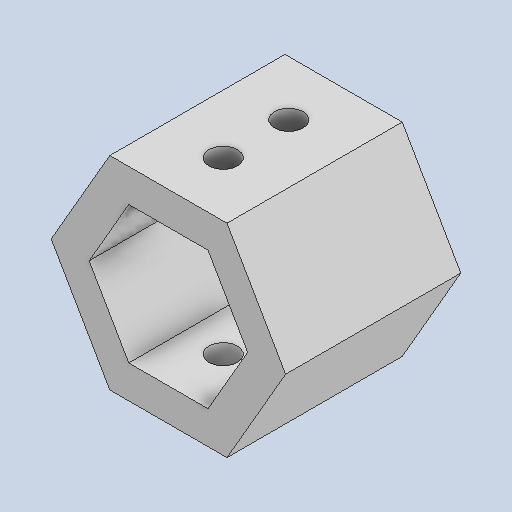
# Autodesk Inventor part: hombro_nuevo
Saved by Autodesk Inventor 2022 (Build 260153000, 153)
## iProperties
Created: 2022-03-10
Part Number: hombro_nuevo
Material: Generic
Document SubType Name: Modeling
Designer: katha
Density: 1 g/cm^3
Appearance: Default
Author: katha
Autodesk Inventor part; units mm, degrees
ref_plane "YZ Plane" through (0, 0, 0) normal (1, 0, 0) x (0, 1, 0)
ref_plane "XZ Plane" through (0, 0, 0) normal (0, 1, 0) x (-1, 0, 0)
ref_plane "XY Plane" through (0, 0, 0) normal (0, 0, 1) x (1, 0, 0)
sketch "Sketch4" plane through (0, 0, 0) normal (0, 0, 1) x (1, 0, 0)
  circle A0 centre (0, 0) radius 3.1 construction
  line L0 (0, 0) -> (3.1, 0) construction
  line L1 (0, 0) -> (1.55, 2.6847) construction
  line L2 (0, 0) -> (-1.55, 2.6847) construction
  line L3 (0, 0) -> (-3.1, 0) construction
  line L4 (0, 0) -> (-1.55, -2.6847) construction
  line L5 (0, 0) -> (1.55, -2.6847) construction
  line L6 (-1.55, 2.6847) -> (1.55, 2.6847) construction
  line L7 (1.55, 2.6847) -> (3.1, 0) construction
  line L8 (3.1, 0) -> (1.55, -2.6847) construction
  line L9 (1.55, -2.6847) -> (-1.55, -2.6847) construction
  line L10 (-1.55, -2.6847) -> (-3.1, 0) construction
  line L11 (-3.1, 0) -> (-1.55, 2.6847) construction
  line L12 (3.6196, 0) -> (1.8098, 3.1347)
  line L13 (1.8098, 3.1347) -> (-1.8098, 3.1347)
  line L14 (-1.8098, 3.1347) -> (-3.6196, 0)
  line L15 (-3.6196, 0) -> (-1.8098, -3.1347)
  line L16 (-1.8098, -3.1347) -> (1.8098, -3.1347)
  line L17 (1.8098, -3.1347) -> (3.6196, 0)
  line L18 (2.6758, 4.6347) -> (5.3517, 0)
  line L19 (5.3517, 0) -> (2.6758, -4.6347)
  line L20 (2.6758, -4.6347) -> (-2.6758, -4.6347)
  line L21 (-2.6758, -4.6347) -> (-5.3517, 0)
  line L22 (-5.3517, 0) -> (-2.6758, 4.6347)
  line L23 (-2.6758, 4.6347) -> (2.6758, 4.6347)
  dimension "d8" = 6.2
  dimension "d11" = 360
  dimension "d13" = 0.45
  dimension "d14" = 1.5
  constraints: 48 end point, 3 coincident, 3 horizontal, 3 parallel, 1 horizontal alignment, 29 other
  measures "d13" distance between parallel lines of L7 L12
  measures "d14" distance between parallel lines of L12 L18
extrude "Extrusion3" add sketch "Sketch4" along normal blind 8
sketch "Sketch5" plane through (-2.6758, 4.6347, 0) normal (0, 1, 0) x (1, 0, 0)
  line L0 (5.3517, 0) -> (0, 0) projected
  line L1 (0, 0) -> (0, -8) projected
  line L2 (5.3517, -8) -> (0, -8) projected
  line L3 (5.3517, 0) -> (5.3517, -8) projected
  circle A0 centre (2.6758, -5.5) radius 0.65
  circle A1 centre (2.6758, -2.5) radius 0.65
  line L4 (5.3517, -8) -> (0, -8) projected
  point P0 (2.6758, 0)
  point P1 (2.6758, -8)
  point P2 (2.6758, -8)
  dimension "d17" = 1.3
  dimension "d18" = 2.5
  dimension "d19" = 2.5
  constraints: 2 centre point, 2 midpoint, 2 vertical alignment, 1 equal radius
  measures "d17" diameter of A0
  measures "d18" distance of point (2.676, -8) A0.centre
  measures "d19" distance of point (2.676, 0) A1.centre
extrude "Extrusion4" cut sketch "Sketch5" against normal blind 10 contours A0 | A1
body "Solid2"
